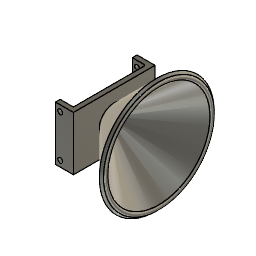
FemaleDrone (Autodesk Fusion 360 archive; units mm, degrees)
design "Female Connector"
Autodesk Fusion 360 part; units mm, degrees
sketch "Sketch1" plane through (0, 0, 0) normal (0, 1, 0) x (1, 0, 0)
  line L0 (7.5, -22.5) -> (-7.5, -22.5)
  line L1 (-7.5, -22.5) -> (-7.5, 22.5)
  line L2 (-7.5, 22.5) -> (7.5, 22.5)
  line L3 (7.5, 22.5) -> (7.5, -22.5)
  line L4 (7.5, -22.5) -> (-7.5, 22.5) construction
  line L5 (-7.5, -22.5) -> (7.5, 22.5) construction
  dimension "d1" = 45
  dimension "d2" = 15
  constraint horizontal L0
  constraint perpendicular L0 L1
  constraint parallel L0 L2
  constraint parallel L1 L3
  constraint coincident L4 origin
  constraint coincident L5 origin
  measures "d1" distance of L0.end L1.end
  measures "d2" distance of L0.start L0.end
extrude "Extrude1" add sketch "Sketch1" along normal blind 4
sketch "Sketch2" plane through (0, 4, 0) normal (0, 1, 0) x (-1, 0, 0)
  line L0 (-7.5, -22.5) -> (7.5, -22.5)
  line L1 (7.5, -22.5) -> (7.5, 22.5)
  line L2 (7.5, 22.5) -> (-7.5, 22.5)
  line L3 (-7.5, 22.5) -> (-7.5, -22.5)
  line L4 (-7.5, 22.5) -> (-3.5, 22.5)
  line L5 (-3.5, 22.5) -> (-3.5, -22.5)
  line L6 (-3.5, -22.5) -> (-7.5, -22.5)
  line L7 (-7.5, -22.5) -> (-7.5, 22.5)
  dimension "d9" = 4
  constraint horizontal L4
  constraint vertical L5
  constraint horizontal L6
  constraint vertical L7
  constraint coincident L0 L5.end
  constraint coincident L2.end L3.start
  measures "d9" distance of L2.end L4.end
extrude "Extrude2" add sketch "Sketch2" along normal blind 64 contours L0 L2 L3 L4 L5 L6 L7
sketch "Sketch3" plane through (3.5, 0, 0) normal (-1, 0, 0) x (0, -1, 0)
  line L0 (-4, -22.5) -> (-4, 22.5)
  line L1 (-4, 22.5) -> (-68, 22.5)
  line L2 (-68, 22.5) -> (-68, -22.5)
  line L3 (-68, -22.5) -> (-4, -22.5)
  line L4 (-68, 22.5) -> (-64, 22.5)
  line L5 (-64, 22.5) -> (-64, -22.5)
  line L6 (-64, -22.5) -> (-68, -22.5)
  line L7 (-68, -22.5) -> (-68, 22.5)
  dimension "d12" = 4
  constraint horizontal L4
  constraint vertical L5
  constraint horizontal L6
  constraint vertical L7
  constraint coincident L3 L5.end
  constraint coincident L1.end L2.start
  measures "d12" distance of L1.end L4.end
extrude "Extrude3" add sketch "Sketch3" along normal blind 11 contours L1 L2 L3 L4 L5 L6 L7
sketch "Sketch4" plane through (3.5, 0, 0) normal (-1, 0, 0) x (0, -1, 0)
  line L0 (-64, 22.5) -> (-64, -22.5)
  line L1 (-64, -22.5) -> (-4, -22.5)
  line L2 (-4, -22.5) -> (-4, 22.5)
  line L3 (-4, 22.5) -> (-64, 22.5)
  line L4 (-60, 22.5) -> (-56, 22.5)
  line L5 (-56, 22.5) -> (-56, -22.5)
  line L6 (-56, -22.5) -> (-60, -22.5)
  line L7 (-60, -22.5) -> (-60, 22.5)
  line L8 (-34, -22.5) -> (-34, 22.5) construction
  line L9 (-8, 22.5) -> (-12, 22.5)
  line L10 (-8, -22.5) -> (-8, 22.5)
  line L11 (-12, 22.5) -> (-12, -22.5)
  line L12 (-12, -22.5) -> (-8, -22.5)
  dimension "d15" = 4
  dimension "d16" = 4
  constraint horizontal L4
  constraint vertical L5
  constraint horizontal L6
  constraint vertical L7
  constraint coincident L1 L5.end
  constraint coincident L3 L4.start
  constraint midpoint L1 L8.start
  constraint midpoint L3 L8.end
  constraint symmetric L4.start L8 L9.start
  constraint symmetric L4.end L8 L9.end
  constraint symmetric L5.end L8 L11.end
  constraint symmetric L6.end L8 L10.start
  measures "d15" distance of L5.end L6.end
  measures "d16" distance of L0 L7
sketch "Sketch5" plane through (0, 68, 0) normal (0, 1, 0) x (-1, 0, 0)
  line L0 (-7.5, -22.5) -> (7.5, -22.5)
  line L1 (7.5, -22.5) -> (7.5, 22.5)
  line L2 (7.5, 22.5) -> (-7.5, 22.5)
  line L3 (-7.5, 22.5) -> (-7.5, -22.5)
  circle A0 centre (3.5, 17.4201) radius 2
  circle A1 centre (3.5, -17.5799) radius 2
  line L4 (3.5, -17.5799) -> (3.5, 17.4201) construction
  point P0 (3.5, -0.0799)
  dimension "d19" = 4
  dimension "d20" = 4
  dimension "d21" = 35
  dimension "d22" = 4
  constraint midpoint L4 P0
  constraint vertical L4
  constraint coincident A0.centre L4.end
  constraint coincident A1.centre L4.start
  measures "d19" diameter of A0
  measures "d20" diameter of A1
  measures "d21" distance of A1.centre A0.centre
  measures "d22" distance of L1 L4
extrude "Extrude5" cut sketch "Sketch5" against normal through all contours A0 | A1
ref_plane "WorkPlane1" through (0, 34, 0) normal (0, 1, 0) x (0, 0, 1)
sketch "Sketch6" plane through (0, 34, 0) normal (0, 1, 0) x (1, 0, 0)
  line L0 (7.5, -12.5) -> (42.8553, -47.8553)
  line L1 (7.5, 22.5) -> (7.5, -22.5)
  line L2 (7.5, 12.5) -> (7.5, -12.5) construction
  line L3 (7.5, 0) -> (0, 0)
  line L4 (42.8553, -47.8553) -> (44.6231, -46.0876)
  line L5 (44.6231, -42.552) -> (7.5, -5.4289)
  arc A0 (44.6231, -46.0876) -> (44.6231, -42.552) centre (42.8553, -44.3198) ccw
  point P0 (7.5, 0)
  point P1 (46.3909, -44.3198)
  dimension "d25" = 50
  dimension "d26" = 25
  dimension "d27" = 135
  dimension "d29" = 5
  dimension "d30" = 2.5
  constraint coincident L0.start L1
  constraint midpoint L2 P0
  constraint coincident L1 P0
  constraint parallel L1 L2
  constraint coincident L0.start L2.end
  constraint coincident P0 L3.start
  constraint coincident L3.end origin
  constraint horizontal L3
  constraint perpendicular L0 L4
  constraint coincident L2 L5.end
  constraint parallel L0 L5
  constraint coincident P1 L5
  constraint coincident P1 L4
  constraint tangent L5 A0
  constraint tangent L4 A0
  measures "d25" distance of L0.start L0.end
  measures "d26" distance of L2.start L0.start
  measures "d27" angle of L0 L2
  measures "d29" distance of L0.end P1
  measures "d30" radius of A0
revolve "Revolve1" add sketch "Sketch6" angle 360 about axis through (7.5, 34, 0) along (-1, 0, 0)
equation "d10 = 56 mm + 8 mm"
equation "d24 = -( 68 / 2 ) * 1 mm"

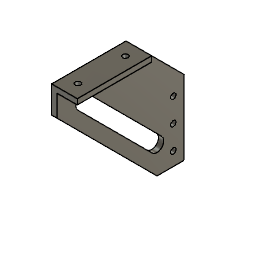
design "DockingMechanismBracketL"
Autodesk Fusion 360 part; units mm, degrees
sketch "Sketch4" plane through (0, 0, 0) normal (1, 0, 0) x (0, 1, 0)
  line L0 (-93.8909, 93.8909) -> (-38.8909, 93.8909)
  line L1 (-38.8909, 93.8909) -> (0, 55)
  line L2 (0, 55) -> (0, 0)
  line L3 (0, 0) -> (-20, 0)
  line L4 (-93.8909, 93.8909) -> (-93.8909, 73.8909)
  line L5 (-93.8909, 73.8909) -> (-20, 0)
  line L6 (-16.4645, 23.5355) -> (-71.4645, 78.5355)
  arc A0 (-71.4645, 78.5355) -> (-78.5355, 71.4645) centre (-75, 75) ccw
  line L7 (-78.5355, 71.4645) -> (-23.5355, 16.4645)
  arc A1 (-23.5355, 16.4645) -> (-16.4645, 23.5355) centre (-20, 20) ccw
  line L8 (-20, 20) -> (-75, 75) construction
  circle A2 centre (-8, 10) radius 2
  circle A3 centre (-8, 45) radius 2
  line L9 (-8, 45) -> (-8, 10) construction
  line L10 (0, 27.5) -> (-8, 27.5) construction
  circle A4 centre (-8, 27.5) radius 2
  dimension "d15" = 55
  dimension "d16" = 135
  dimension "d17" = 55
  dimension "d18" = 55
  dimension "d19" = 20
  dimension "d20" = 20
  dimension "d21" = 10
  dimension "d22" = 4
  dimension "d23" = 4
  dimension "d24" = 8
  dimension "d25" = 35
  dimension "d35" = 4
  constraint horizontal L0
  constraint vertical L2
  constraint perpendicular L2 L3
  constraint vertical L4
  constraint tangent L6 A0
  constraint tangent A0 L7
  constraint parallel L6 L7
  constraint tangent L7 A1
  constraint tangent L6 A1
  constraint coincident A3.centre L9.start
  constraint coincident A2.centre L9.end
  constraint vertical L9
  constraint midpoint L2 L10.start
  constraint midpoint L9 L10.end
  constraint perpendicular L2 L10
  constraint coincident L0.start L4.start
  constraint coincident L2.end L3.start
  constraint coincident L10.end A4.centre
  measures "d15" distance of L0.start L0.end
  measures "d16" angle of L0 L1
  measures "d17" distance of L0.end L1.end
  measures "d18" distance of L1.end L2.end
  measures "d19" distance of L2.end L3.end
  measures "d20" distance of L0.start L4.end
  measures "d21" diameter of A0
  measures "d22" diameter of A2
  measures "d23" diameter of A3
  measures "d24" distance of L2 L9
  measures "d25" distance of A3.centre A2.centre
  measures "d35" diameter of A4
extrude "Extrude1" add sketch "Sketch4" along normal blind 4
sketch "Sketch5" plane through (0, 0, 93.8909) normal (0, 0, 1) x (-1, 0, 0)
  line L0 (0, 38.8909) -> (0, 93.8909)
  line L1 (0, 93.8909) -> (-4, 93.8909)
  line L2 (-4, 93.8909) -> (-4, 38.8909)
  line L3 (-4, 38.8909) -> (0, 38.8909)
  line L4 (0, 93.8909) -> (-19, 93.8909)
  line L5 (-19, 93.8909) -> (-19, 38.8909)
  line L6 (-19, 38.8909) -> (0, 38.8909)
  line L7 (0, 38.8909) -> (0, 93.8909)
  circle A0 centre (-9.5, 83.8909) radius 2
  circle A1 centre (-9.5, 48.8909) radius 2
  line L8 (-9.5, 83.8909) -> (-9.5, 48.8909) construction
  line L9 (-9.5, 66.3909) -> (0, 66.3909) construction
  line L10 (-9.5, 48.8909) -> (-9.5, 38.8909) construction
  dimension "d28" = 55
  dimension "d30" = 4
  dimension "d31" = 4
  dimension "d32" = 35
  dimension "d36" = 19
  constraint horizontal L4
  constraint vertical L5
  constraint horizontal L6
  constraint vertical L7
  constraint coincident L0.end L1.start
  constraint coincident A0.centre L8.start
  constraint coincident A1.centre L8.end
  constraint midpoint L8 L9.start
  constraint midpoint L7 L9.end
  constraint perpendicular L7 L9
  constraint midpoint L6 L10.end
  constraint perpendicular L6 L10
  constraint vertical L8
  measures "d28" distance of L0.end L0.start
  measures "d30" diameter of A0
  measures "d31" diameter of A1
  measures "d32" vertical distance of A0.centre A1.centre
  measures "d36" distance of L0.end L4.end
extrude "Extrude3" add sketch "Sketch5" against normal blind 4 contours L2 L4 L5 L6

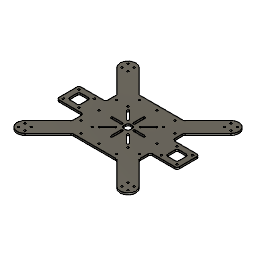
design "DroneBase"
Autodesk Fusion 360 part; units mm, degrees
sketch "Sketch1" plane through (0, 0, 0) normal (0, 0, 1) x (1, 0, 0)
  line L0 (0, 0) -> (0, 75) construction
  line L1 (0, 0) -> (75, 0) construction
  line L2 (-50, 75) -> (50, 75)
  line L3 (75, -50) -> (75, 50)
  line L4 (0, 0) -> (0, -75) construction
  line L5 (0, 0) -> (-75, 0) construction
  line L6 (-50, -75) -> (50, -75)
  line L7 (-75, -50) -> (-75, 50)
  line L8 (-50, 75) -> (-103.033, 128.033)
  line L9 (-75, 50) -> (-128.033, 103.033)
  arc A0 (-103.033, 128.033) -> (-128.033, 103.033) centre (-115.533, 115.533) ccw
  line L10 (50, 75) -> (103.033, 128.033)
  line L11 (75, 50) -> (128.033, 103.033)
  arc A1 (128.033, 103.033) -> (103.033, 128.033) centre (115.533, 115.533) ccw
  line L12 (75, -50) -> (128.033, -103.033)
  line L13 (50, -75) -> (103.033, -128.033)
  arc A2 (103.033, -128.033) -> (128.033, -103.033) centre (115.533, -115.533) ccw
  line L14 (-50, -75) -> (-103.033, -128.033)
  line L15 (-75, -50) -> (-128.033, -103.033)
  arc A3 (-128.033, -103.033) -> (-103.033, -128.033) centre (-115.533, -115.533) ccw
  line L16 (-75, 25) -> (-75, -25)
  line L17 (-75, -25) -> (-135, -25)
  line L18 (-135, -25) -> (-135, 25)
  line L19 (-135, 25) -> (-75, 25)
  line L20 (-135, 0) -> (-75, 0) construction
  line L21 (75, -25) -> (135, -25)
  line L22 (135, -25) -> (135, 25)
  line L23 (135, 25) -> (75, 25)
  dimension "d1" = 75
  dimension "d2" = 75
  dimension "d3" = 75
  dimension "d4" = 75
  dimension "d5" = 100
  dimension "d6" = 135
  dimension "d7" = 75
  dimension "d10" = 135
  dimension "d11" = 135
  dimension "d12" = 135
  dimension "d13" = 60
  dimension "d14" = 50
  constraint coincident L0.start L1.start
  constraint vertical L0
  constraint perpendicular L0 L1
  constraint midpoint L0.end L2
  constraint perpendicular L0 L2
  constraint midpoint L1.end L3
  constraint perpendicular L1 L3
  constraint perpendicular L1 L4
  constraint perpendicular L4 L5
  constraint midpoint L4.end L6
  constraint perpendicular L4 L6
  constraint midpoint L5.end L7
  constraint perpendicular L5 L7
  constraint equal L2 L7
  constraint equal L2 L3
  constraint equal L3 L6
  constraint parallel L8 L9
  constraint tangent L8 A0
  constraint equal L8 L9
  constraint equal L8 L10
  constraint equal L10 L11
  constraint parallel L10 L11
  constraint tangent L10 A1
  constraint parallel L12 L13
  constraint equal L8 L12
  constraint equal L12 L13
  constraint tangent L12 A2
  constraint parallel L14 L15
  constraint equal L14 L15
  constraint equal L8 L14
  constraint tangent L15 A3
  constraint perpendicular L16 L17
  constraint parallel L16 L18
  constraint parallel L17 L19
  constraint coincident L7 L16.end
  constraint perpendicular L5 L16
  constraint midpoint L18 L20.start
  constraint midpoint L16 L5.end
  constraint coincident L5.end L20.end
  constraint symmetric L0 L16.start L23.end
  constraint symmetric L0 L16.end L21.start
  constraint symmetric L0 L17.end L21.end
  constraint symmetric L0 L18.end L22.end
  measures "d1" distance of L0.start L0.end
  measures "d2" distance of L0.start L1.end
  measures "d3" distance of L0.start L4.end
  measures "d4" distance of L0.start L5.end
  measures "d5" distance of L7.start L7.end
  measures "d6" angle of L2 L8
  measures "d7" distance of L2.start L8.end
  measures "d10" angle of L2 L10
  measures "d11" angle of L6 L13
  measures "d12" angle of L6 L14
  measures "d13" distance of L16.start L18.end
  measures "d14" distance of L17.end L18.end
  measures "d27" distance of L3.end
extrude "Extrude1" add sketch "Sketch1" along normal blind 4
sketch "Sketch2" plane through (0, 0, 4) normal (0, 0, 1) x (-1, 0, 0)
  line L0 (-75, 50) -> (-75, 25)
  line L1 (-75, 25) -> (-135, 25)
  line L2 (-135, 25) -> (-135, -25)
  line L3 (-135, -25) -> (-75, -25)
  line L4 (-75, -25) -> (-75, -50)
  line L5 (-75, -50) -> (-128.033, -103.033)
  arc A0 (-128.033, -103.033) -> (-103.033, -128.033) centre (-115.533, -115.533) ccw
  line L6 (-103.033, -128.033) -> (-50, -75)
  line L7 (-50, -75) -> (50, -75)
  line L8 (50, -75) -> (103.033, -128.033)
  arc A1 (103.033, -128.033) -> (128.033, -103.033) centre (115.533, -115.533) ccw
  line L9 (128.033, -103.033) -> (75, -50)
  line L10 (75, -50) -> (75, -25)
  line L11 (75, -25) -> (135, -25)
  line L12 (135, -25) -> (135, 25)
  line L13 (135, 25) -> (75, 25)
  line L14 (75, 25) -> (75, 50)
  line L15 (75, 50) -> (128.033, 103.033)
  arc A2 (128.033, 103.033) -> (103.033, 128.033) centre (115.533, 115.533) ccw
  line L16 (103.033, 128.033) -> (50, 75)
  line L17 (50, 75) -> (-50, 75)
  line L18 (-50, 75) -> (-103.033, 128.033)
  arc A3 (-103.033, 128.033) -> (-128.033, 103.033) centre (-115.533, 115.533) ccw
  line L19 (-128.033, 103.033) -> (-75, 50)
  line L20 (92.5, -17.5) -> (127.5, -17.5) construction
  line L21 (127.5, -17.5) -> (127.5, 17.5) construction
  line L22 (127.5, 17.5) -> (92.5, 17.5) construction
  line L23 (92.5, 17.5) -> (92.5, -17.5) construction
  line L24 (92.5, -17.5) -> (127.5, 17.5) construction
  line L25 (127.5, -17.5) -> (92.5, 17.5) construction
  circle A4 centre (127.5, -17.5) radius 2
  circle A5 centre (92.5, -17.5) radius 2
  circle A6 centre (127.5, 17.5) radius 2
  circle A7 centre (92.5, 17.5) radius 2
  line L26 (101.5, -12.5) -> (118.5, -12.5)
  line L27 (122.5, -8.5) -> (122.5, 8.5)
  line L28 (118.5, 12.5) -> (101.5, 12.5)
  line L29 (97.5, 8.5) -> (97.5, -8.5)
  line L30 (97.5, -12.5) -> (122.5, 12.5) construction
  line L31 (122.5, -12.5) -> (97.5, 12.5) construction
  arc A8 (118.5, -12.5) -> (122.5, -8.5) centre (118.5, -8.5) ccw
  arc A9 (122.5, 8.5) -> (118.5, 12.5) centre (118.5, 8.5) ccw
  arc A10 (101.5, 12.5) -> (97.5, 8.5) centre (101.5, 8.5) ccw
  arc A11 (97.5, -8.5) -> (101.5, -12.5) centre (101.5, -8.5) ccw
  line L32 (0, 75) -> (0, -75) construction
  line L33 (-122.5, -8.5) -> (-122.5, 8.5)
  arc A12 (-122.5, -8.5) -> (-118.5, -12.5) centre (-118.5, -8.5) ccw
  line L34 (-101.5, -12.5) -> (-118.5, -12.5)
  arc A13 (-101.5, -12.5) -> (-97.5, -8.5) centre (-101.5, -8.5) ccw
  line L35 (-97.5, 8.5) -> (-97.5, -8.5)
  line L36 (-118.5, 12.5) -> (-101.5, 12.5)
  arc A14 (-97.5, 8.5) -> (-101.5, 12.5) centre (-101.5, 8.5) ccw
  arc A15 (-118.5, 12.5) -> (-122.5, 8.5) centre (-118.5, 8.5) ccw
  circle A16 centre (-127.5, 17.5) radius 2
  circle A17 centre (-127.5, -17.5) radius 2
  circle A18 centre (-92.5, -17.5) radius 2
  circle A19 centre (-92.5, 17.5) radius 2
  line L37 (-40, -40) -> (40, -40) construction
  line L38 (40, -40) -> (40, 40) construction
  line L39 (40, 40) -> (-40, 40) construction
  line L40 (-40, 40) -> (-40, -40) construction
  line L41 (-40, -40) -> (40, 40) construction
  line L42 (40, -40) -> (-40, 40) construction
  circle A20 centre (40, -40) radius 2
  circle A21 centre (-40, -40) radius 2
  line L43 (-75, 0) -> (75, 0) construction
  circle A22 centre (40, 40) radius 2
  circle A23 centre (-40, 40) radius 2
  line L44 (-30.4056, -33.234) -> (-12.7279, -15.5563)
  arc A24 (-12.7279, -15.5563) -> (-15.5563, -12.7279) centre (-14.1421, -14.1421) ccw
  line L45 (-15.5563, -12.7279) -> (-33.234, -30.4056)
  arc A25 (-33.234, -30.4056) -> (-30.4056, -33.234) centre (-31.8198, -31.8198) ccw
  line L46 (-31.8198, -31.8198) -> (-14.1421, -14.1421) construction
  line L47 (-30.4056, 33.234) -> (-12.7279, 15.5563)
  arc A26 (-15.5563, 12.7279) -> (-12.7279, 15.5563) centre (-14.1421, 14.1421) ccw
  line L48 (-15.5563, 12.7279) -> (-33.234, 30.4056)
  arc A27 (-30.4056, 33.234) -> (-33.234, 30.4056) centre (-31.8198, 31.8198) ccw
  arc A28 (15.5563, -12.7279) -> (12.7279, -15.5563) centre (14.1421, -14.1421) ccw
  line L49 (15.5563, -12.7279) -> (33.234, -30.4056)
  arc A29 (30.4056, -33.234) -> (33.234, -30.4056) centre (31.8198, -31.8198) ccw
  line L50 (30.4056, -33.234) -> (12.7279, -15.5563)
  arc A30 (12.7279, 15.5563) -> (15.5563, 12.7279) centre (14.1421, 14.1421) ccw
  line L51 (15.5563, 12.7279) -> (33.234, 30.4056)
  line L52 (30.4056, 33.234) -> (12.7279, 15.5563)
  arc A31 (33.234, 30.4056) -> (30.4056, 33.234) centre (31.8198, 31.8198) ccw
  line L53 (75, 40) -> (40, 40) construction
  line L54 (40, 40) -> (40, 75) construction
  circle A32 centre (65, 40) radius 2
  circle A33 centre (40, 65) radius 2
  circle A34 centre (-40, 65) radius 2
  circle A35 centre (-65, 40) radius 2
  circle A36 centre (65, -40) radius 2
  circle A37 centre (40, -65) radius 2
  circle A38 centre (-40, -65) radius 2
  circle A39 centre (-65, -40) radius 2
  line L55 (-2.5, -7.5) -> (2.5, -7.5)
  line L56 (7.5, -2.5) -> (7.5, 2.5)
  line L57 (2.5, 7.5) -> (-2.5, 7.5)
  line L58 (-7.5, 2.5) -> (-7.5, -2.5)
  line L59 (-7.5, -7.5) -> (7.5, 7.5) construction
  line L60 (7.5, -7.5) -> (-7.5, 7.5) construction
  arc A40 (2.5, -7.5) -> (7.5, -2.5) centre (2.5, -2.5) ccw
  arc A41 (7.5, 2.5) -> (2.5, 7.5) centre (2.5, 2.5) ccw
  arc A42 (-2.5, 7.5) -> (-7.5, 2.5) centre (-2.5, 2.5) ccw
  arc A43 (-7.5, -2.5) -> (-2.5, -7.5) centre (-2.5, -2.5) ccw
  line L61 (14, -2) -> (36.5, -2)
  arc A44 (36.5, -2) -> (36.5, 2) centre (36.5, 0) ccw
  line L62 (36.5, 2) -> (14, 2)
  arc A45 (14, 2) -> (14, -2) centre (14, 0) ccw
  line L63 (14, 0) -> (36.5, 0) construction
  line L64 (-14, -2) -> (-36.5, -2)
  line L65 (-36.5, 2) -> (-14, 2)
  arc A46 (-14, -2) -> (-14, 2) centre (-14, 0) ccw
  arc A47 (-36.5, 2) -> (-36.5, -2) centre (-36.5, 0) ccw
  line L66 (-2, 36.5) -> (-2, 14)
  line L67 (2, 14) -> (2, 36.5)
  arc A48 (2, 36.5) -> (-2, 36.5) centre (0, 36.5) ccw
  arc A49 (-2, 14) -> (2, 14) centre (0, 14) ccw
  line L68 (-2, -36.5) -> (-2, -14)
  arc A50 (2, -14) -> (-2, -14) centre (0, -14) ccw
  line L69 (2, -14) -> (2, -36.5)
  arc A51 (-2, -36.5) -> (2, -36.5) centre (0, -36.5) ccw
  line L70 (-36.5, -2) -> (-14, -2)
  line L71 (-14, 2) -> (-36.5, 2)
  arc A52 (-36.5, 2) -> (-36.5, -2) centre (-36.5, 0) ccw
  arc A53 (-14, -2) -> (-14, 2) centre (-14, 0) ccw
  line L72 (36.5, -2) -> (14, -2)
  arc A54 (14, 2) -> (14, -2) centre (14, 0) ccw
  line L73 (14, 2) -> (36.5, 2)
  arc A55 (36.5, -2) -> (36.5, 2) centre (36.5, 0) ccw
  line L74 (2, -36.5) -> (2, -14)
  line L75 (-2, -14) -> (-2, -36.5)
  arc A56 (-2, -36.5) -> (2, -36.5) centre (0, -36.5) ccw
  arc A57 (2, -14) -> (-2, -14) centre (0, -14) ccw
  line L76 (2, 36.5) -> (2, 14)
  arc A58 (-2, 14) -> (2, 14) centre (0, 14) ccw
  line L77 (-2, 14) -> (-2, 36.5)
  arc A59 (2, 36.5) -> (-2, 36.5) centre (0, 36.5) ccw
  circle A60 centre (0, 65) radius 2
  circle A61 centre (-65, 0) radius 2
  circle A62 centre (0, -65) radius 2
  circle A63 centre (65, 0) radius 2
  point P0 (110, 0)
  point P1 (110, 0)
  dimension "d17" = 35
  dimension "d18" = 35
  dimension "d19" = 25
  dimension "d20" = 25
  dimension "d21" = 4
  dimension "d25" = 25
  dimension "d26" = 4
  dimension "d27" = 80
  dimension "d28" = 80
  dimension "d29" = 4
  dimension "d30" = 25
  dimension "d31" = 4
  dimension "d32" = 25
  dimension "d33" = 20
  dimension "d44" = 75
  dimension "d45" = 4
  dimension "d46" = 4
  dimension "d47" = 25
  dimension "d48" = 25
  dimension "d49" = 15
  dimension "d50" = 15
  dimension "d51" = 5
  dimension "d52" = 4
  dimension "d53" = 14
  dimension "d54" = 22.5
  dimension "d56" = 360
  dimension "d57" = 4
  dimension "d59" = 360
  constraint horizontal L20
  constraint perpendicular L20 L21
  constraint parallel L20 L22
  constraint parallel L21 L23
  constraint coincident L24 P1
  constraint coincident L25 P1
  constraint coincident L20.end L21.start
  constraint coincident L20.start L23.end
  constraint coincident L21.end L22.start
  constraint coincident L22.end L23.start
  constraint horizontal L26
  constraint perpendicular L26 L27
  constraint parallel L26 L28
  constraint parallel L27 L29
  constraint coincident L30 P1
  constraint coincident L31 P1
  constraint coincident P1 P0
  constraint coincident L31.start L26
  constraint coincident L31.start L27
  constraint tangent L26 A8
  constraint tangent L27 A8
  constraint coincident L30.end L27
  constraint coincident L30.end L28
  constraint tangent L27 A9
  constraint tangent L28 A9
  constraint equal A8 A9
  constraint coincident L31.end L28
  constraint coincident L31.end L29
  constraint tangent L28 A10
  constraint tangent L29 A10
  constraint equal A8 A10
  constraint coincident L30.start L29
  constraint coincident L30.start L26
  constraint tangent L29 A11
  constraint tangent L26 A11
  constraint equal A8 A11
  constraint midpoint L32 origin
  constraint coincident L7 L32.end
  constraint perpendicular L7 L32
  constraint symmetric A4 L32 A17
  constraint symmetric A5 L32 A18
  constraint symmetric A6 L32 A16
  constraint symmetric A7 L32 A19
  constraint symmetric L26.end L32 A12.end
  constraint symmetric L27.start L32 L33.start
  constraint symmetric A8 L32 A12
  constraint symmetric L27.end L32 L33.end
  constraint symmetric L28.start L32 L36.start
  constraint symmetric A9 L32 A15
  constraint symmetric L28.end L32 L36.end
  constraint symmetric L29.start L32 L35.start
  constraint symmetric A10 L32 A14
  constraint symmetric L29.end L32 A13.end
  constraint symmetric L26.start L32 L34.start
  constraint symmetric A11 L32 A13
  constraint horizontal L37
  constraint perpendicular L37 L38
  constraint parallel L37 L39
  constraint parallel L38 L40
  constraint coincident L41 origin
  constraint coincident L42 origin
  constraint coincident L37.end L38.start
  constraint symmetric L32 A20 A21
  constraint perpendicular L23 L43
  constraint symmetric A20 L43 A22
  constraint symmetric A21 L43 A23
  constraint equal A4 A5
  constraint equal A5 A7
  constraint equal A6 A7
  constraint tangent L44 A24
  constraint tangent A24 L45
  constraint parallel L44 L45
  constraint tangent L45 A25
  constraint tangent L44 A25
  constraint coincident L41 A24.centre
  constraint parallel L41 L46
  constraint symmetric L43 L44.start L47.start
  constraint symmetric L43 L44.end L47.end
  constraint symmetric L43 A24.end A26.start
  constraint symmetric L43 L45.end L48.end
  constraint symmetric L43 A24 A26
  constraint symmetric L43 A25 A27
  constraint symmetric L32 L44.start A29.start
  constraint symmetric L32 L44.end A28.end
  constraint symmetric L32 A24.end A28.start
  constraint symmetric L32 L45.end L49.end
  constraint symmetric L32 A24 A28
  constraint symmetric L32 A25 A29
  constraint symmetric L32 L47.start L52.start
  constraint symmetric L32 L47.end A30.start
  constraint symmetric L32 A26.start A30.end
  constraint symmetric L32 A26 A30
  constraint symmetric L32 L48.end L51.end
  constraint symmetric L32 A27 A31
  constraint coincident L14 L53.start
  constraint coincident L38.end L39.start
  constraint perpendicular L14 L53
  constraint coincident L17 L54.end
  constraint perpendicular L17 L54
  constraint coincident L53 A32.centre
  constraint coincident L54 A33.centre
  constraint symmetric L32 A32 A35
  constraint symmetric L32 A33 A34
  constraint symmetric L43 A32 A36
  constraint symmetric L43 A33 A37
  constraint symmetric L43 A34 A38
  constraint symmetric L43 A35 A39
  constraint horizontal L55
  constraint perpendicular L55 L56
  constraint parallel L55 L57
  constraint parallel L56 L58
  constraint coincident L59 origin
  constraint coincident L60 origin
  constraint coincident L60.start L55
  constraint coincident L60.start L56
  constraint tangent L55 A40
  constraint tangent L56 A40
  constraint coincident L59.end L56
  constraint coincident L59.end L57
  constraint tangent L56 A41
  constraint tangent L57 A41
  constraint equal A40 A41
  constraint coincident L60.end L57
  constraint coincident L60.end L58
  constraint tangent L57 A42
  constraint tangent L58 A42
  constraint equal A40 A42
  constraint coincident L59.start L58
  constraint coincident L59.start L55
  constraint tangent L58 A43
  constraint tangent L55 A43
  constraint equal A40 A43
  constraint tangent L61 A44
  constraint tangent A44 L62
  constraint parallel L61 L62
  constraint tangent L62 A45
  constraint tangent L61 A45
  constraint coincident L43 A44.centre
  constraint parallel L43 L63
  constraint symmetric L32 L61.start L64.start
  constraint symmetric L32 L61.end L64.end
  constraint symmetric L32 A44.end L65.start
  constraint symmetric L32 L62.end L65.end
  constraint symmetric L32 A44 A47
  constraint symmetric L32 A45 A46
  constraint coincident L32 A60.centre
  measures "d17" distance of L20.end L21.end
  measures "d18" distance of L20.start L20.end
  measures "d19" distance of L12 P1
  measures "d20" distance of L13 P1
  measures "d21" diameter of A4
  measures "d25" distance of L31.start L30.end
  measures "d26" radius of A8
  measures "d27" distance of L37.end L38.end
  measures "d28" distance of L38.end L39.end
  measures "d29" diameter of A20
  measures "d30" distance of L27 L29
  measures "d31" diameter of A24
  measures "d32" distance of A24.end L45.end
  measures "d33" distance of origin A24.centre
  measures "d44" distance of L7 L43
  measures "d45" diameter of A32
  measures "d46" diameter of A33
  measures "d47" distance of L38.end A33.centre
  measures "d48" distance of L38.end A32.centre
  measures "d49" distance of L60.start L59.end
  measures "d50" distance of L59.end L60.end
  measures "d51" radius of A40
  measures "d52" diameter of A44
  measures "d53" distance of origin A45.centre
  measures "d54" distance of L61.start L61.end
  measures "d57" diameter of A60
extrude "Extrude2" cut sketch "Sketch2" against normal through all contours A4 | A5 | A6 | A7 | L26 L27 L28 L29 A8 A9 A10 A11 | L33 A12 L34 A13 L35 L36 A14 A15 | A16 | A17 | A18 | A19 | A20 | A21 | A22 | A23 | L44 A24 L45 A25 | L47 A26 L48 A27 | A28 L49 A29 L50 | A30 L51 L52 A31 | A32 | A33 | A34 | A35 | A36 | A37 | A38 | A39 | L55 L56 L57 L58 A40 A41 A42 A43 | L61 A44 L62 A45 L72 A54 L73 A55 | L64 L65 A46 A47 L70 L71 A52 A53 | L66 L67 A48 A49 L76 A58 L77 A59 | L68 A50 L69 A51 L74 L75 A56 A57 | A60 | A61 | A62 | A63
fillet "Fillet1" radius 5 16 edges at (75, -50, 2) (75, -25, 2) (135, -25, 2) (135, 25, 2) (75, 25, 2) (75, 50, 2) (50, 75, 2) (-50, 75, 2) (-75, 25, 2) (-75, 50, 2) (-135, 25, 2) (-135, -25, 2) (-75, -25, 2) (-75, -50, 2) (-50, -75, 2) (50, -75, 2)
sketch "Sketch3" plane through (0, 0, 4) normal (0, 0, 1) x (-1, 0, 0)
  circle A0 centre (127.5, 17.5) radius 2
  circle A1 centre (92.5, 17.5) radius 2
  line L0 (33.234, 30.4056) -> (15.5563, 12.7279)
  arc A2 (12.7279, 15.5563) -> (15.5563, 12.7279) centre (14.1421, 14.1421) ccw
  line L1 (12.7279, 15.5563) -> (30.4056, 33.234)
  arc A3 (33.234, 30.4056) -> (30.4056, 33.234) centre (31.8198, 31.8198) ccw
  circle A4 centre (-40, -40) radius 2
  line L2 (-101.5, -12.5) -> (-118.5, -12.5)
  arc A5 (-122.5, -8.5) -> (-118.5, -12.5) centre (-118.5, -8.5) ccw
  line L3 (-122.5, -8.5) -> (-122.5, 8.5)
  arc A6 (-118.5, 12.5) -> (-122.5, 8.5) centre (-118.5, 8.5) ccw
  line L4 (-118.5, 12.5) -> (-101.5, 12.5)
  arc A7 (-97.5, 8.5) -> (-101.5, 12.5) centre (-101.5, 8.5) ccw
  line L5 (-97.5, 8.5) -> (-97.5, -8.5)
  arc A8 (-101.5, -12.5) -> (-97.5, -8.5) centre (-101.5, -8.5) ccw
  circle A9 centre (-127.5, 17.5) radius 2
  line L6 (-33.234, -30.4056) -> (-15.5563, -12.7279)
  arc A10 (-12.7279, -15.5563) -> (-15.5563, -12.7279) centre (-14.1421, -14.1421) ccw
  line L7 (-12.7279, -15.5563) -> (-30.4056, -33.234)
  arc A11 (-33.234, -30.4056) -> (-30.4056, -33.234) centre (-31.8198, -31.8198) ccw
  line L8 (-15.5563, 12.7279) -> (-33.234, 30.4056)
  arc A12 (-30.4056, 33.234) -> (-33.234, 30.4056) centre (-31.8198, 31.8198) ccw
  line L9 (-30.4056, 33.234) -> (-12.7279, 15.5563)
  arc A13 (-15.5563, 12.7279) -> (-12.7279, 15.5563) centre (-14.1421, 14.1421) ccw
  line L10 (101.5, 12.5) -> (118.5, 12.5)
  arc A14 (122.5, 8.5) -> (118.5, 12.5) centre (118.5, 8.5) ccw
  line L11 (122.5, 8.5) -> (122.5, -8.5)
  arc A15 (118.5, -12.5) -> (122.5, -8.5) centre (118.5, -8.5) ccw
  line L12 (118.5, -12.5) -> (101.5, -12.5)
  arc A16 (97.5, -8.5) -> (101.5, -12.5) centre (101.5, -8.5) ccw
  line L13 (97.5, -8.5) -> (97.5, 8.5)
  arc A17 (101.5, 12.5) -> (97.5, 8.5) centre (101.5, 8.5) ccw
  circle A18 centre (127.5, -17.5) radius 2
  circle A19 centre (40, 40) radius 2
  circle A20 centre (40, -40) radius 2
  circle A21 centre (-92.5, -17.5) radius 2
  circle A22 centre (-127.5, -17.5) radius 2
  circle A23 centre (-92.5, 17.5) radius 2
  line L14 (15.5563, -12.7279) -> (33.234, -30.4056)
  arc A24 (30.4056, -33.234) -> (33.234, -30.4056) centre (31.8198, -31.8198) ccw
  line L15 (30.4056, -33.234) -> (12.7279, -15.5563)
  arc A25 (15.5563, -12.7279) -> (12.7279, -15.5563) centre (14.1421, -14.1421) ccw
  circle A26 centre (-40, 40) radius 2
  circle A27 centre (92.5, -17.5) radius 2
  arc A28 (135, 20) -> (130, 25) centre (130, 20) ccw
  line L16 (130, 25) -> (80, 25)
  arc A29 (75, 30) -> (80, 25) centre (80, 30) ccw
  line L17 (75, 30) -> (75, 47.9289)
  arc A30 (76.4645, 51.4645) -> (75, 47.9289) centre (80, 47.9289) ccw
  line L18 (76.4645, 51.4645) -> (128.033, 103.033)
  arc A31 (128.033, 103.033) -> (103.033, 128.033) centre (115.533, 115.533) ccw
  line L19 (103.033, 128.033) -> (51.4645, 76.4645)
  arc A32 (47.9289, 75) -> (51.4645, 76.4645) centre (47.9289, 80) ccw
  line L20 (47.9289, 75) -> (-47.9289, 75)
  arc A33 (-51.4645, 76.4645) -> (-47.9289, 75) centre (-47.9289, 80) ccw
  line L21 (-51.4645, 76.4645) -> (-103.033, 128.033)
  arc A34 (-103.033, 128.033) -> (-128.033, 103.033) centre (-115.533, 115.533) ccw
  line L22 (-128.033, 103.033) -> (-76.4645, 51.4645)
  arc A35 (-75, 47.9289) -> (-76.4645, 51.4645) centre (-80, 47.9289) ccw
  line L23 (-75, 47.9289) -> (-75, 30)
  arc A36 (-80, 25) -> (-75, 30) centre (-80, 30) ccw
  line L24 (-80, 25) -> (-130, 25)
  arc A37 (-130, 25) -> (-135, 20) centre (-130, 20) ccw
  line L25 (-135, 20) -> (-135, -20)
  arc A38 (-135, -20) -> (-130, -25) centre (-130, -20) ccw
  line L26 (-130, -25) -> (-80, -25)
  arc A39 (-75, -30) -> (-80, -25) centre (-80, -30) ccw
  line L27 (-75, -30) -> (-75, -47.9289)
  arc A40 (-76.4645, -51.4645) -> (-75, -47.9289) centre (-80, -47.9289) ccw
  line L28 (-76.4645, -51.4645) -> (-128.033, -103.033)
  arc A41 (-128.033, -103.033) -> (-103.033, -128.033) centre (-115.533, -115.533) ccw
  line L29 (-103.033, -128.033) -> (-51.4645, -76.4645)
  arc A42 (-47.9289, -75) -> (-51.4645, -76.4645) centre (-47.9289, -80) ccw
  line L30 (-47.9289, -75) -> (47.9289, -75)
  arc A43 (51.4645, -76.4645) -> (47.9289, -75) centre (47.9289, -80) ccw
  line L31 (51.4645, -76.4645) -> (103.033, -128.033)
  arc A44 (103.033, -128.033) -> (128.033, -103.033) centre (115.533, -115.533) ccw
  line L32 (128.033, -103.033) -> (76.4645, -51.4645)
  arc A45 (75, -47.9289) -> (76.4645, -51.4645) centre (80, -47.9289) ccw
  line L33 (75, -47.9289) -> (75, -30)
  arc A46 (80, -25) -> (75, -30) centre (80, -30) ccw
  line L34 (80, -25) -> (130, -25)
  arc A47 (130, -25) -> (135, -20) centre (130, -20) ccw
  line L35 (135, -20) -> (135, 20)
  line L36 (108.4613, 122.6035) -> (122.6047, 108.4625) construction
  line L37 (122.6035, 122.6047) -> (108.4625, 108.4613) construction
  line L38 (128.033, 103.033) -> (103.033, 128.033) construction
  line L39 (115.533, 115.533) -> (128.033, 128.033) construction
  circle A48 centre (122.6047, 108.4625) radius 2
  circle A49 centre (122.6035, 122.6047) radius 2
  circle A50 centre (108.4613, 122.6035) radius 2
  circle A51 centre (108.4625, 108.4613) radius 2
  line L40 (75, 0) -> (-75, 0) construction
  line L41 (0, 75) -> (0, -75) construction
  circle A52 centre (-122.6047, 108.4625) radius 2
  circle A53 centre (-108.4625, 108.4613) radius 2
  circle A54 centre (-122.6035, 122.6047) radius 2
  circle A55 centre (-108.4613, 122.6035) radius 2
  circle A56 centre (-122.6035, -122.6047) radius 2
  circle A57 centre (-108.4613, -122.6035) radius 2
  circle A58 centre (-108.4625, -108.4613) radius 2
  circle A59 centre (-122.6047, -108.4625) radius 2
  circle A60 centre (122.6035, -122.6047) radius 2
  circle A61 centre (122.6047, -108.4625) radius 2
  circle A62 centre (108.4625, -108.4613) radius 2
  circle A63 centre (108.4613, -122.6035) radius 2
  circle A64 centre (65, -40) radius 2
  circle A65 centre (-65, 40) radius 2
  circle A66 centre (65, 40) radius 2
  circle A67 centre (-65, -40) radius 2
  circle A68 centre (40, -65) radius 2
  circle A69 centre (-40, 65) radius 2
  circle A70 centre (40, 65) radius 2
  circle A71 centre (-40, -65) radius 2
  line L42 (-2.5, 7.5) -> (2.5, 7.5)
  arc A72 (7.5, 2.5) -> (2.5, 7.5) centre (2.5, 2.5) ccw
  line L43 (7.5, 2.5) -> (7.5, -2.5)
  arc A73 (2.5, -7.5) -> (7.5, -2.5) centre (2.5, -2.5) ccw
  line L44 (2.5, -7.5) -> (-2.5, -7.5)
  arc A74 (-7.5, -2.5) -> (-2.5, -7.5) centre (-2.5, -2.5) ccw
  line L45 (-7.5, -2.5) -> (-7.5, 2.5)
  arc A75 (-2.5, 7.5) -> (-7.5, 2.5) centre (-2.5, 2.5) ccw
  line L46 (-14, -2) -> (-36.5, -2)
  arc A76 (-36.5, 2) -> (-36.5, -2) centre (-36.5, 0) ccw
  line L47 (-36.5, 2) -> (-14, 2)
  arc A77 (-14, -2) -> (-14, 2) centre (-14, 0) ccw
  line L48 (2, -14) -> (2, -36.5)
  arc A78 (-2, -36.5) -> (2, -36.5) centre (0, -36.5) ccw
  line L49 (-2, -36.5) -> (-2, -14)
  arc A79 (2, -14) -> (-2, -14) centre (0, -14) ccw
  line L50 (-2, 14) -> (-2, 36.5)
  arc A80 (2, 36.5) -> (-2, 36.5) centre (0, 36.5) ccw
  line L51 (2, 36.5) -> (2, 14)
  arc A81 (-2, 14) -> (2, 14) centre (0, 14) ccw
  line L52 (14, 2) -> (36.5, 2)
  arc A82 (36.5, -2) -> (36.5, 2) centre (36.5, 0) ccw
  line L53 (36.5, -2) -> (14, -2)
  arc A83 (14, 2) -> (14, -2) centre (14, 0) ccw
  circle A84 centre (0, -65) radius 2
  circle A85 centre (-65, 0) radius 2
  circle A86 centre (65, 0) radius 2
  circle A87 centre (0, 65) radius 2
  point P0 (115.533, 115.533)
  point P1 (115.533, 115.533)
  dimension "d37" = 20
  dimension "d38" = 20
  dimension "d39" = 4
  dimension "d40" = 4
  dimension "d41" = 4
  dimension "d42" = 4
  constraint midpoint L36 P1
  constraint midpoint L37 P1
  constraint coincident P1 P0
  constraint perpendicular L36 L37
  constraint coincident L18.end A31.start
  constraint coincident A31.end L19.start
  constraint midpoint A31 L39.end
  constraint coincident L36.end A48.centre
  constraint coincident L37.start A49.centre
  constraint coincident L36.start A50.centre
  constraint coincident L37.end A51.centre
  constraint horizontal L40
  constraint midpoint L20 L41.start
  constraint midpoint L30 L41.end
  constraint symmetric A48 L41 A52
  constraint symmetric A49 L41 A54
  constraint symmetric A50 L41 A55
  constraint symmetric A51 L41 A53
  constraint symmetric A48 L40 A61
  constraint symmetric A49 L40 A60
  constraint symmetric A50 L40 A63
  constraint symmetric A51 L40 A62
  constraint symmetric L40 A52 A59
  constraint symmetric L40 A53 A58
  constraint symmetric L40 A54 A56
  constraint symmetric L40 A55 A57
  measures "d37" distance of L37.start L37.end
  measures "d38" distance of L36.start L36.end
  measures "d39" diameter of A48
  measures "d40" diameter of A49
  measures "d41" diameter of A50
  measures "d42" diameter of A51
extrude "Extrude3" cut sketch "Sketch3" against normal through all contours A48 | A49 | A50 | A51 | A52 | A53 | A54 | A55 | A56 | A57 | A58 | A59 | A60 | A61 | A62 | A63

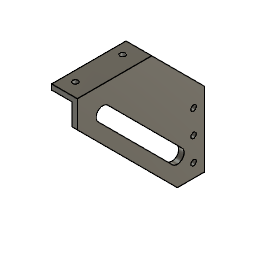
design "DockingMechanismBracketR"
Autodesk Fusion 360 part; units mm, degrees
sketch "Sketch4" plane through (0, 0, 0) normal (1, 0, 0) x (0, 1, 0)
  line L0 (-93.8909, 93.8909) -> (-38.8909, 93.8909)
  line L1 (-38.8909, 93.8909) -> (0, 55)
  line L2 (0, 55) -> (0, 0)
  line L3 (0, 0) -> (-20, 0)
  line L4 (-93.8909, 93.8909) -> (-93.8909, 73.8909)
  line L5 (-93.8909, 73.8909) -> (-20, 0)
  line L6 (-16.4645, 23.5355) -> (-71.4645, 78.5355)
  arc A0 (-71.4645, 78.5355) -> (-78.5355, 71.4645) centre (-75, 75) ccw
  line L7 (-78.5355, 71.4645) -> (-23.5355, 16.4645)
  arc A1 (-23.5355, 16.4645) -> (-16.4645, 23.5355) centre (-20, 20) ccw
  line L8 (-20, 20) -> (-75, 75) construction
  circle A2 centre (-8, 10) radius 2
  circle A3 centre (-8, 45) radius 2
  line L9 (-8, 45) -> (-8, 10) construction
  line L10 (0, 27.5) -> (-8, 27.5) construction
  circle A4 centre (-8, 27.5) radius 2
  dimension "d15" = 55
  dimension "d16" = 135
  dimension "d17" = 55
  dimension "d18" = 55
  dimension "d19" = 20
  dimension "d20" = 20
  dimension "d21" = 10
  dimension "d22" = 4
  dimension "d23" = 4
  dimension "d24" = 8
  dimension "d25" = 35
  dimension "d35" = 4
  constraint horizontal L0
  constraint vertical L2
  constraint perpendicular L2 L3
  constraint vertical L4
  constraint tangent L6 A0
  constraint tangent A0 L7
  constraint parallel L6 L7
  constraint tangent L7 A1
  constraint tangent L6 A1
  constraint coincident A3.centre L9.start
  constraint coincident A2.centre L9.end
  constraint vertical L9
  constraint midpoint L2 L10.start
  constraint midpoint L9 L10.end
  constraint perpendicular L2 L10
  constraint coincident L0.start L4.start
  constraint coincident L2.end L3.start
  constraint coincident L10.end A4.centre
  measures "d15" distance of L0.start L0.end
  measures "d16" angle of L0 L1
  measures "d17" distance of L0.end L1.end
  measures "d18" distance of L1.end L2.end
  measures "d19" distance of L2.end L3.end
  measures "d20" distance of L0.start L4.end
  measures "d21" diameter of A0
  measures "d22" diameter of A2
  measures "d23" diameter of A3
  measures "d24" distance of L2 L9
  measures "d25" distance of A3.centre A2.centre
  measures "d35" diameter of A4
extrude "Extrude1" add sketch "Sketch4" along normal blind 4
sketch "Sketch5" plane through (0, 0, 93.8909) normal (0, 0, 1) x (-1, 0, 0)
  line L0 (0, 38.8909) -> (0, 93.8909)
  line L1 (0, 93.8909) -> (-4, 93.8909)
  line L2 (-4, 93.8909) -> (-4, 38.8909)
  line L3 (-4, 38.8909) -> (0, 38.8909)
  line L4 (0, 93.8909) -> (15, 93.8909)
  line L5 (15, 93.8909) -> (15, 38.8909)
  line L6 (15, 38.8909) -> (0, 38.8909)
  line L7 (0, 38.8909) -> (0, 93.8909)
  circle A0 centre (7.5, 83.8909) radius 2
  circle A1 centre (7.5, 48.8909) radius 2
  line L8 (7.5, 83.8909) -> (7.5, 48.8909) construction
  line L9 (7.5, 66.3909) -> (0, 66.3909) construction
  line L10 (7.5, 48.8909) -> (7.5, 38.8909) construction
  dimension "d28" = 55
  dimension "d29" = 15
  dimension "d30" = 4
  dimension "d31" = 4
  dimension "d32" = 35
  constraint horizontal L4
  constraint vertical L5
  constraint horizontal L6
  constraint vertical L7
  constraint coincident L0.end L1.start
  constraint coincident A0.centre L8.start
  constraint coincident A1.centre L8.end
  constraint midpoint L8 L9.start
  constraint midpoint L7 L9.end
  constraint perpendicular L7 L9
  constraint midpoint L6 L10.end
  constraint perpendicular L6 L10
  constraint vertical L8
  measures "d28" distance of L0.end L0.start
  measures "d29" distance of L0.end L4.end
  measures "d30" diameter of A0
  measures "d31" diameter of A1
  measures "d32" vertical distance of A0.centre A1.centre
extrude "Extrude2" add sketch "Sketch5" against normal blind 4 contours L0 L4 L5 L6 L7
